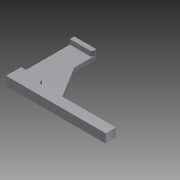
# Autodesk Inventor part: Tirador
Saved by Autodesk Inventor 2011 (Build 150239000, 239)
## iProperties
Created: 2014-08-04
Part Number: Tirador
Material: Por defecto
Document SubType Name: Chapa
Designer: amatiasq
Density: 1 g/cm^3
Sheet Metal Rule: Por defecto_mm
Author: amatiasq
Autodesk Inventor part; units mm, degrees
ref_plane "YZ Plane" through (0, 0, 0) normal (1, 0, 0) x (0, 1, 0)
ref_plane "XZ Plane" through (0, 0, 0) normal (0, 1, 0) x (-1, 0, 0)
ref_plane "XY Plane" through (0, 0, 0) normal (0, 0, 1) x (1, 0, 0)
sketch "Boceto1" plane through (0, 0, 0) normal (0, 0, 1) x (1, 0, 0)
  line L0 (0, 0) -> (0, 30.8)
  line L1 (0, 30.8) -> (10, 30.8)
  line L2 (10, 30.8) -> (10, 20.8)
  line L3 (0, 0) -> (45, 0)
  line L4 (45, 0) -> (45, 4.6)
  line L5 (45, 4.6) -> (20, 4.6)
  line L6 (20, 4.6) -> (10, 20.8)
  dimension "d0" = 30.8
  dimension "d1" = 10
  dimension "d2" = 10
  dimension "d3" = 45
  dimension "d4" = 4.6
  dimension "d5" = 25
  constraints: 14 end point, 3 perpendicular, 2 parallel, 1 vertical
  measures "d0" distance of L0.start L0.end
  measures "d1" distance of L0.end L1.end
  measures "d2" distance of L1.end L2.end
  measures "d3" distance of L0.start L3.end
  measures "d4" distance of L3.end L4.end
  measures "d5" distance of L4.end L5.end
extrude "Extrusión1" add sketch "Boceto1" along normal blind 1.8
sketch "Boceto2" plane through (0, 0, 1.8) normal (0, 0, 1) x (1, 0, 0)
  line L0 (0, 30.8) -> (10, 30.8) projected
  line L1 (0, 0) -> (0, 30.8) projected
  line L2 (45, 0) -> (0, 0) projected
  line L3 (45, 4.6) -> (45, 0) projected
  line L4 (20, 4.6) -> (45, 4.6) projected
  line L5 (10, 30.8) -> (10, 20.8) projected
  line L6 (20, 4.6) -> (10.5, 4.6)
  line L7 (0, 6.8) -> (9.5, 6.8)
  line L8 (9.5, 6.8) -> (10.5, 4.6)
  line L9 (0, 28.8) -> (9.5, 28.8)
  line L10 (9.5, 28.8) -> (10, 29.9002)
  line L11 (9.5, 28.8) -> (10.7085, 28.8) construction
  dimension "d8" = 9.5
  dimension "d9" = 9.5
  dimension "d10" = 9.5
  dimension "d11" = 65.56
  constraints: 12 end point, 3 point on line, 2 parallel, 1 equal length, 1 horizontal, 1 perpendicular
  measures "d8" distance of L4.start L6.end
  measures "d9" distance of L7.start L7.end
  measures "d10" distance of L9.start L9.end
  measures "d11" angle of L11 L10
extrude "Extrusión2" add sketch "Boceto2" along normal blind 2.2
equation "\"Radio_pliegue\" = Grosor"
equation "\"Anchura_desahogo_plegado\" = Grosor"
equation "\"Profundidad_desahogo_plegado\" = 0.5 * Grosor"
equation "\"Tamaño_destalonado\" = 4 * Grosor"
equation "\"Remanente_mínimo\" = 2 * Grosor"
equation "\"Radiodetransición\" = Radio_pliegue"
equation "\"Tamaño_de_radio_de_Jacobi\" = Radio_pliegue"
equation "\"TamañoSeparación\" = Grosor"
equation "\"Grosor\" = 0.5"
